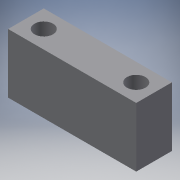
# Autodesk Inventor part: Abstandhalter_MPU
Saved by Autodesk Inventor 2018 (Build 220112000, 112)
## iProperties
Created: 2018-01-29
Part Number: Abstandhalter_MPU
Material: Generisch
Document SubType Name: Modeling
Designer: Chris
Density: 1 g/cm^3
Appearance: Vorgabe
Author: Chris
Autodesk Inventor part; units mm, degrees
ref_plane "YZ Plane" through (0, 0, 0) normal (1, 0, 0) x (0, 1, 0)
ref_plane "XZ Plane" through (0, 0, 0) normal (0, 1, 0) x (-1, 0, 0)
ref_plane "XY Plane" through (0, 0, 0) normal (0, 0, 1) x (1, 0, 0)
sketch "Skizze1" plane through (0, 0, 0) normal (0, 0, 1) x (1, 0, 0)
  circle A0 centre (7.7787, 5.2388) radius 1.5558 projected
  circle A1 centre (-7.7788, 5.2387) radius 1.5558 projected
  line L0 (10.5537, 7.874) -> (10.5537, -7.874) projected
  line L1 (-10.5537, -7.874) -> (-10.5537, 7.874) projected
  line L2 (-10.5537, 7.874) -> (10.5537, 7.874) projected
  line L3 (10.5537, -7.874) -> (-10.5537, -7.874) projected
  line L4 (-10.7788, 8.2387) -> (10.7787, 8.2387)
  line L5 (10.7787, 8.2387) -> (10.7787, 2.2388)
  line L6 (10.7787, 2.2388) -> (-10.7788, 2.2388)
  line L7 (-10.7788, 2.2388) -> (-10.7788, 8.2387)
  point P0 (0, 0)
  dimension "d2" = 3
  dimension "d3" = 3
  dimension "d4" = 3
  dimension "d5" = 3
  constraints: 8 end point, 2 parallel, 1 horizontal, 1 perpendicular
  measures "d2" distance from line of L4 A1.centre
  measures "d3" distance from line of A1.centre L7
  measures "d4" distance from line of L5 A0.centre
  measures "d5" distance from line of L6 A0.centre
extrude "Extrusion1" add sketch "Skizze1" along normal blind 10 contours L2 L1 L6 L7 L4 L5 L0 | L0 L6 L1 L2
